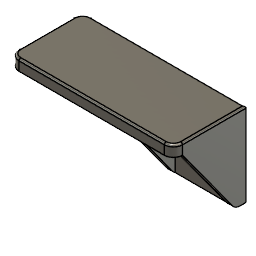
Docking Station Assembly (Autodesk Fusion 360 archive; units mm, degrees)
design "Ramp fitting"
Autodesk Fusion 360 part; units mm, degrees
sketch "Sketch1" plane through (0, 0, 0) normal (0, 1, 0) x (1, 0, 0)
  line L0 (0, 0) -> (36, 0)
  line L1 (36, 0) -> (36, 6)
  line L2 (36, 6) -> (0, 6)
  line L3 (0, 6) -> (0, 0)
  dimension "d1" = 36
  dimension "d2" = 6
  constraint horizontal L0
  constraint vertical L1
  constraint horizontal L2
  constraint vertical L3
  constraint coincident L0.start L3.end
  measures "d1" distance of L1.end L2.end
  measures "d2" distance of L0.end L1.end
extrude "Extrude1" add sketch "Sketch1" along normal blind 40
sketch "Sketch2" plane through (0, 0, 0) normal (0, 0, 1) x (1, 0, 0)
  line L0 (0, 0) -> (36, 0)
  line L1 (36, 0) -> (36, 40)
  line L2 (36, 40) -> (0, 40)
  line L3 (0, 40) -> (0, 0)
  line L4 (18, 40) -> (18, 0) construction
  line L5 (36, 20) -> (0, 20) construction
  line L6 (7.8571, 40) -> (7.8571, 0) construction
  line L7 (32.8571, 40) -> (32.8571, 0) construction
  line L8 (8, 17.4) -> (28, 17.4)
  arc A0 (28, 17.4) -> (28, 22.6) centre (28, 20) ccw
  line L9 (28, 22.6) -> (8, 22.6)
  arc A1 (8, 22.6) -> (8, 17.4) centre (8, 20) ccw
  line L10 (8, 20) -> (28, 20) construction
  dimension "d33" = 5.2
  dimension "d34" = 10
  dimension "d35" = 10
  dimension "d37" = 20
  constraint midpoint L2 L4.start
  constraint midpoint L0 L4.end
  constraint midpoint L1 L5.start
  constraint midpoint L3 L5.end
  constraint coincident L2 L6.start
  constraint coincident L0 L6.end
  constraint perpendicular L0 L6
  constraint coincident L2 L7.start
  constraint coincident L0 L7.end
  constraint perpendicular L0 L7
  constraint tangent L8 A0
  constraint tangent A0 L9
  constraint parallel L8 L9
  constraint tangent L9 A1
  constraint tangent L8 A1
  constraint perpendicular L7 L10
  measures "d33" diameter of A0
  measures "d34" distance of L4 A1.centre
  measures "d35" distance of L4 A0.centre
  measures "d37" distance of L2 A1.centre
extrude "Extrude2" cut sketch "Sketch2" against normal up to surface (6 mm away) contours L8 A0 L9 A1
sketch "Sketch4" plane through (36, 0, 0) normal (1, 0, 0) x (0, 0, -1)
  line L0 (0, 0) -> (6, 0)
  line L1 (6, 0) -> (6, 40)
  line L2 (6, 40) -> (0, 40)
  line L3 (0, 40) -> (0, 0)
  line L4 (6, 40) -> (-34, 40)
  line L5 (-34, 40) -> (-34, 46)
  line L6 (-34, 46) -> (6, 46)
  line L7 (6, 46) -> (6, 40)
  dimension "d12" = 40
  dimension "d13" = 6
  constraint horizontal L4
  constraint vertical L5
  constraint horizontal L6
  constraint vertical L7
  constraint coincident L1.end L2.start
  measures "d12" distance of L1.end L4.end
  measures "d13" distance of L1.end L6.end
extrude "Extrude4" add sketch "Sketch4" against normal blind 90 contours L2 L4 L5 L6 L7
fillet "Fillet1" [suppressed]
fillet "Fillet2" radius 5 3 edges at (-54, 43, -6) (-54, 43, 34) (36, 43, 34)
fillet "Fillet3" radius 1 1 faces at (6, 46, 7.3333)
sketch "Sketch5" plane through (36, 0, 0) normal (1, 0, 0) x (0, 0, -1)
  line L0 (6, 45) -> (-29, 45)
  line L1 (-29, 45) -> (-29, 40)
  line L2 (-29, 40) -> (0, 40)
  line L3 (0, 40) -> (0, 0)
  line L4 (0, 0) -> (6, 0)
  line L5 (6, 0) -> (6, 45)
  line L6 (0, 0) -> (-29, 40)
  constraint coincident L3.end L4.start
  constraint coincident L1.end L2.start
extrude "Extrude5" add sketch "Sketch5" against normal blind 3 contours L2 L3 L6
ref_plane "WorkPlane1" through (18, 22.5, 11.5) normal (1, 0, 0) x (0, 0, -1)
mirror "Mirror1" about plane through (18, 22.5, 11.5) normal (1, 0, 0) of "Extrude5"
fillet "Fillet4" radius 5 2 edges at (34.5, 0, 0) (1.5, 0, 0)

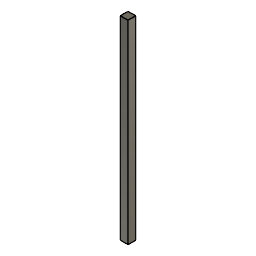
design "40 x 40 x 1000 Pole"
Autodesk Fusion 360 part; units mm, degrees
sketch "Sketch2" plane through (0, 0, 0) normal (0, 0, 1) x (1, 0, 0)
  line L0 (20, 20) -> (-20, 20)
  line L1 (-20, 20) -> (-20, -20)
  line L2 (-20, -20) -> (20, -20)
  line L3 (20, -20) -> (20, 20)
  line L4 (20, 20) -> (-20, -20) construction
  line L5 (-20, 20) -> (20, -20) construction
  dimension "d1" = 40
  dimension "d2" = 40
  constraint horizontal L0
  constraint perpendicular L0 L1
  constraint parallel L0 L2
  constraint parallel L1 L3
  constraint coincident L4 origin
  constraint coincident L5 origin
  measures "d1" distance of L1.end L2.end
  measures "d2" distance of L0.end L1.end
extrude "Extrude1" add sketch "Sketch2" along normal blind 1000

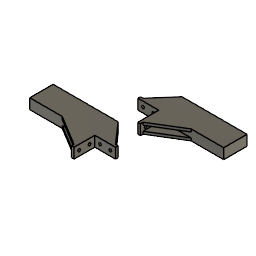
design "spring stopper"
Autodesk Fusion 360 part; units mm, degrees
sketch "Sketch1" plane through (0, 0, 0) normal (0, 0, 1) x (1, 0, 0)
  line L0 (0, 0) -> (125, 0)
  line L1 (125, 0) -> (125, 45)
  line L2 (125, 45) -> (0, 45)
  line L3 (0, 45) -> (0, 0)
  line L4 (0, 0) -> (-40, 0)
  line L5 (-40, 0) -> (-40, -40)
  line L6 (-40, -40) -> (0, -40)
  line L7 (0, -40) -> (0, 0)
  line L8 (-40, 0) -> (-40, 5)
  line L9 (-40, 5) -> (0, 5)
  line L10 (0, -40) -> (5, -40)
  line L11 (5, -40) -> (5, 0)
  line L12 (62.5, 0) -> (5, -35)
  line L13 (-35, 5) -> (0, 45)
  dimension "d1" = 125
  dimension "d2" = 45
  dimension "d3" = 40
  dimension "d4" = 40
  dimension "d6" = 5
  dimension "d9" = 5
  dimension "d13" = 5
  dimension "d14" = 5
  constraint horizontal L0
  constraint vertical L1
  constraint horizontal L2
  constraint vertical L3
  constraint coincident L0.start L3.end
  constraint horizontal L4
  constraint vertical L5
  constraint horizontal L6
  constraint vertical L7
  constraint perpendicular L4 L8
  constraint coincident L3 L9.end
  constraint perpendicular L3 L9
  constraint perpendicular L7 L10
  constraint coincident L0 L11.end
  constraint perpendicular L0 L11
  constraint midpoint L0 L12.start
  constraint coincident L11 L12.end
  constraint coincident L9 L13.start
  measures "d1" distance of L0.start L0.end
  measures "d2" distance of L0.start L2.end
  measures "d3" distance of L0.start L4.end
  measures "d4" distance of L0.start L6.end
  measures "d6" distance of L4.end L8.end
  measures "d9" distance of L6.end L10.end
  measures "d13" distance of L10 L12.end
  measures "d14" distance of L8.end L13.start
extrude "Extrude1" add sketch "Sketch1" along normal blind 20 contours L0 L1 L2 L3 | L3 L4 L8 L9 | L0 L7 L10 L11 makes body 1
extrude "Extrude2" add sketch "Sketch1" along normal blind 5 contours L0 L11 L12 | L3 L9 L13 bodies 1
extrude "Extrude4" add 2 faces at (24.1667, -11.6667, 5) (-11.6667, 18.3333, 5) along direction (0, 0, -1) blind 5 start surface through (0, 0, 20) normal (0, 0, 1) on bodies 1 bodies 1
sketch "Sketch2" plane through (5, 0, 0) normal (1, 0, 0) x (0, 1, 0)
  line L0 (-35, 15) -> (-35, 20)
  line L1 (-35, 20) -> (-40, 20)
  line L2 (-40, 20) -> (-40, 0)
  line L3 (-40, 0) -> (-35, 0)
  line L4 (-35, 0) -> (-35, 5)
  line L5 (-35, 5) -> (0, 5)
  line L6 (0, 5) -> (0, 15)
  line L7 (0, 15) -> (-35, 15)
  line L8 (-40, 10) -> (0, 10) construction
  circle A0 centre (-30, 10) radius 2.6
  circle A1 centre (-10, 10) radius 2.6
  dimension "d24" = 5.2
  dimension "d25" = 5.2
  dimension "d26" = 10
  dimension "d27" = 10
  constraint midpoint L2 L8.start
  constraint midpoint L6 L8.end
  constraint coincident L8 A0.centre
  constraint coincident L8 A1.centre
  measures "d24" diameter of A0
  measures "d25" diameter of A1
  measures "d26" distance of L8.start A0.centre
  measures "d27" distance of L8.end A1.centre
extrude "Extrude5" cut sketch "Sketch2" against normal blind 5 contours A0 | A1 bodies 1
sketch "Sketch3" plane through (0, 5, 0) normal (0, 1, 0) x (-1, 0, 0)
  line L0 (35, 20) -> (35, 15)
  line L1 (35, 15) -> (0, 15)
  line L2 (0, 15) -> (0, 5)
  line L3 (0, 5) -> (35, 5)
  line L4 (35, 5) -> (35, 0)
  line L5 (35, 0) -> (40, 0)
  line L6 (40, 0) -> (40, 20)
  line L7 (40, 20) -> (35, 20)
  line L8 (0, 10) -> (40, 10) construction
  circle A0 centre (10, 10) radius 2.6
  circle A1 centre (30, 10) radius 2.6
  dimension "d30" = 5.2
  dimension "d31" = 5.2
  dimension "d32" = 10
  dimension "d33" = 10
  constraint midpoint L2 L8.start
  constraint midpoint L6 L8.end
  constraint coincident L8 A0.centre
  constraint coincident L8 A1.centre
  measures "d30" diameter of A0
  measures "d31" diameter of A1
  measures "d32" distance of L8.start A0.centre
  measures "d33" distance of L8.end A1.centre
extrude "Extrude6" cut sketch "Sketch3" against normal blind 5 contours A0 | A1 bodies 1
mirror "Mirror1" about plane through (0, 0, 0) normal (1, 0, 0) of bodies 1 makes body 2
move_body "Move1" bodies 2 to x (1, 0, 0) y (0, 1, 0) z (0, 0, 1) at (-47.5192, -75.3246, -27.8054)
